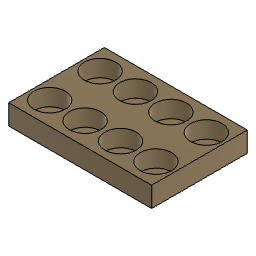
vial_rack v3 (Autodesk Fusion 360 design; units mm, degrees)
Autodesk Fusion 360 part; units mm, degrees
sketch "Sketch1" plane through (0, 0, 0) normal (0, 0, 1) x (1, 0, 0)
  line L0 (63.875, -42.75) -> (-63.875, -42.75)
  line L1 (-63.875, -42.75) -> (-63.875, 42.75)
  line L2 (-63.875, 42.75) -> (63.875, 42.75)
  line L3 (63.875, 42.75) -> (63.875, -42.75)
  line L4 (63.875, -42.75) -> (-63.875, 42.75) construction
  line L5 (-63.875, -42.75) -> (63.875, 42.75) construction
  dimension "d1" = 127.75
  dimension "d2" = 85.5
  constraint horizontal L0
  constraint perpendicular L0 L1
  constraint parallel L0 L2
  constraint parallel L1 L3
  constraint coincident L4 origin
  constraint coincident L5 origin
  measures "d1" distance of L1.end L2.end
  measures "d2" distance of L0.end L1.end
extrude "Extrude1" add sketch "Sketch1" along normal blind 3
sketch "Sketch2" plane through (0, 0, 3) normal (0, 0, 1) x (-1, 0, 0)
  line L0 (-63.875, -42.75) -> (63.875, -42.75)
  line L1 (63.875, -42.75) -> (63.875, 42.75)
  line L2 (63.875, 42.75) -> (-63.875, 42.75)
  line L3 (-63.875, 42.75) -> (-63.875, -42.75)
  line L4 (-63.875, -42.75) -> (-63.875, 42.75)
  line L5 (-63.875, 42.75) -> (63.875, 42.75)
  line L6 (63.875, 42.75) -> (63.875, -42.75)
  line L7 (63.875, -42.75) -> (-63.875, -42.75)
  line L8 (0, 0) -> (47.5, 0) construction
  line L9 (47.5, 0) -> (47.5, -22.5) construction
  circle A0 centre (47.5, -22.5) radius 13.5
  circle A1 centre (47.5, -22.5) radius 14
  circle A2 centre (15.8333, -22.5) radius 14
  circle A3 centre (-15.8333, -22.5) radius 14
  circle A4 centre (-47.5, -22.5) radius 14
  circle A5 centre (47.5, 22.5) radius 14
  circle A6 centre (15.8333, 22.5) radius 14
  circle A7 centre (-15.8333, 22.5) radius 14
  circle A8 centre (-47.5, 22.5) radius 14
  dimension "d5" = 47.5
  dimension "d6" = 22.5
  dimension "d7" = 27
  dimension "d8" = 0.5
  dimension "d15" = -95
  dimension "d16" = 45
  constraint coincident L8.start origin
  constraint parallel L7 L8
  constraint perpendicular L8 L9
  constraint coincident L9.end A0.centre
  measures "d5" distance of L8.start L8.end
  measures "d6" distance of L8.end L9.end
  measures "d7" diameter of A0
extrude "Extrude2" add sketch "Sketch2" along normal blind 15 contours L0 L1 L2 L3 L4 L5 L6 L7
